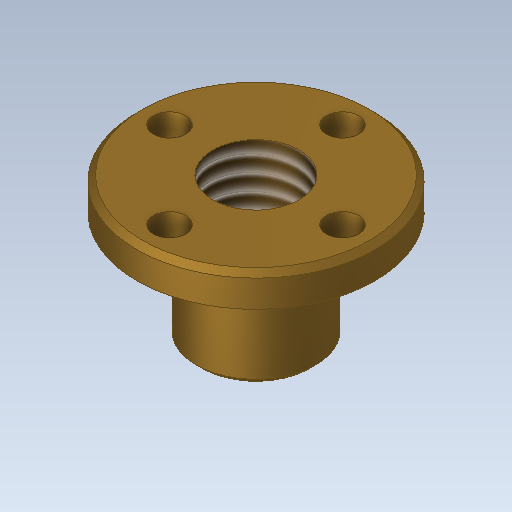
# Autodesk Inventor part: 25_nakrętka trapezowa
Saved by Autodesk Inventor 2020.2 (Build 242310000, 310)
## iProperties
Created: 2017-10-28
Part Number: 25_nakrętka trapezowa
Material: Mosiądz, miękki żółty
Document SubType Name: Modeling
Designer: wojte
Density: 8.47 g/cm^3
Appearance: Mosiądz — satynowy
Author: wojte
Autodesk Inventor part; units mm, degrees
ref_plane "YZ Plane" through (0, 0, 0) normal (1, 0, 0) x (0, 1, 0)
ref_plane "XZ Plane" through (0, 0, 0) normal (0, 1, 0) x (-1, 0, 0)
ref_plane "XY Plane" through (0, 0, 0) normal (0, 0, 1) x (1, 0, 0)
sketch "Szkic1" plane through (0, 0, 0) normal (0, 1, 0) x (-1, 0, 0)
  circle A0 centre (0, 0) radius 5.5
  dimension "d0" = 11
  constraints: 1 centre point, 1 coincident
  measures "d0" diameter of A0
extrude "Wyciągnięcie proste1" add sketch "Szkic1" along normal blind 10
sketch "Szkic2" plane through (0, 10, 0) normal (0, 1, 0) x (1, 0, 0)
  circle A0 centre (0, 0) radius 11
  dimension "d3" = 22
  constraints: 1 centre point, 1 coincident
  measures "d3" diameter of A0
extrude "Wyciągnięcie proste2" add sketch "Szkic2" along normal blind 3
sketch "Szkic3" plane through (0, 13, 0) normal (0, 1, 0) x (1, 0, 0)
  point P0 (0, 0)
  point P1 (-8, 0)
  point P2 (0, -8)
  point P3 (8, 0)
  point P4 (0, 8)
  dimension "d6" = 8
  dimension "d9" = 360
  constraints: 1 horizontal alignment, 5 other
  measures "d6" distance of point (0, 0) point (-8, 0)
hole "Otwór1" at (-8, 13, 0) at (0, 13, 8) at (8, 13, 0) at (0, 13, -8) direction (0, -1, 0) diameter 3 end through all
sketch "Szkic4" plane through (0, 13, 0) normal (0, 1, 0) x (1, 0, 0)
  point P0 (0, 0)
  point P1 (0, 0)
  constraints: 1 coincident
hole "Otwór2" at (0, 13, 0) direction (0, -1, 0) diameter 8 end through all
chamfer "Faza1" distance 0.5 angle 45 2 edges at (-11, 13, 0) (5.5, 0, 0)
thread "Gwint1" size "TR8x1.5" class "7H" standard "ISO Metric Trapezoidal Threads" full length
